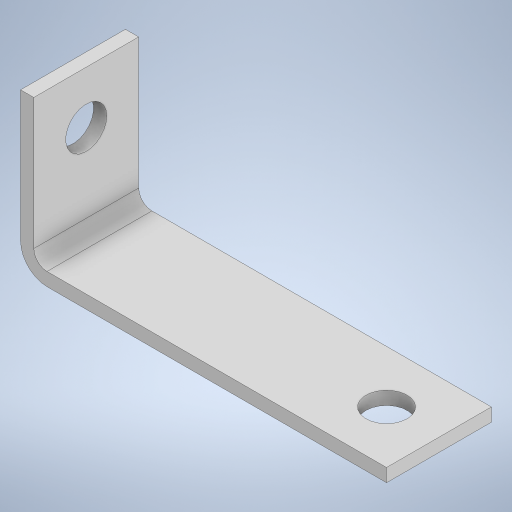
# Autodesk Inventor part: Bracket
Saved by Autodesk Inventor 2023 (Build 270158000, 158)
## iProperties
Created: 2023-10-20
Part Number: Bracket
Material: Generic
Document SubType Name: Modeling
Designer: jackc
Density: 1 g/cm^3
Appearance: Default
Author: jackc
Autodesk Inventor part; units mm, degrees
ref_plane "YZ Plane" through (0, 0, 0) normal (1, 0, 0) x (0, 1, 0)
ref_plane "XZ Plane" through (0, 0, 0) normal (0, 1, 0) x (-1, 0, 0)
ref_plane "XY Plane" through (0, 0, 0) normal (0, 0, 1) x (1, 0, 0)
sketch "Sketch1" plane through (0, 0, 0) normal (0, 0, 1) x (1, 0, 0)
  line L0 (-3.2004, 19.05) -> (-3.2004, 3.2004)
  arc A0 (-3.2004, 3.2004) -> (0, 0) centre (0, 3.2004) ccw
  line L1 (0, 0) -> (41.1226, 0)
  line L2 (41.1226, 0) -> (41.1226, 1.6002)
  line L3 (41.1226, 1.6002) -> (0, 1.6002)
  arc A1 (-1.6002, 3.2004) -> (0, 1.6002) centre (0, 3.2004) ccw
  line L4 (-1.6002, 3.2004) -> (-1.6002, 19.05)
  line L5 (-1.6002, 19.05) -> (-3.2004, 19.05)
  point P0 (0, 0)
  dimension "d0" = 1.6002
  dimension "d1" = 19.05
  dimension "d2" = 44.323
  dimension "d3" = 1.6002
  constraints: 12 end point, 4 perpendicular, 4 point on circle, 4 tangent, 2 centre point, 1 coincident, 1 concentric, 1 horizontal, 1 vertical
  measures "d0" distance of L1.end L2.end
  measures "d1" distance between parallel lines of L1 L5
  measures "d2" distance between parallel lines of L2 L0
  measures "d3" radius of A1
extrude "Extrusion1" add sketch "Sketch1" along normal blind 12.7
sketch "Sketch2" plane through (-1.6002, 3.2004, 0) normal (1, 0, 0) x (0, 0, -1)
  line L0 (0, -3.2004) -> (-12.7, -3.2004) projected
  circle A0 centre (-6.35, 9.4996) radius 2.4892
  line L1 (0, 0) -> (0, 15.8496) projected
  dimension "d6" = 4.9784
  dimension "d7" = 12.7
  dimension "d8" = 6.35
  constraints: 1 centre point
  measures "d6" diameter of A0
  measures "d7" distance from line of L0 A0.centre
  measures "d8" distance from line of L1 A0.centre
sketch "Sketch3" plane through (0, 1.6002, 0) normal (0, 1, 0) x (1, 0, 0)
  circle A0 centre (34.7759, -6.35) radius 2.4892
  line L0 (-3.2004, 0) -> (-3.2004, -12.7) projected
  line L1 (41.1226, -12.7) -> (0, -12.7) projected
  point P0 (0, 0)
  dimension "d9" = 37.9763
  dimension "d10" = 6.35
  dimension "d11" = 4.9784
  constraints: 1 centre point
  measures "d9" distance from line of A0.centre L0
  measures "d10" distance from line of L1 A0.centre
  measures "d11" diameter of A0
extrude "Extrusion2" cut sketch "Sketch2" against normal blind 12.7
extrude "Extrusion3" cut sketch "Sketch3" against normal blind 12.7
equation "\"d3\" = d0"
body "Solid1"
